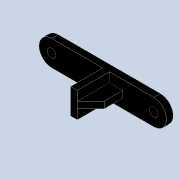
# Autodesk Inventor part: Y Axis Limit Switch Trigger
Saved by Autodesk Inventor 2022 (Build 260153000, 153)
## iProperties
Created: 2021-10-29
Part Number: Y Axis Limit Switch Trigger
Material: Generic
Document SubType Name: Modeling
Designer: Coy
Density: 1 g/cm^3
Appearance: Anodized - Black
Author: Coy
Autodesk Inventor part; units mm, degrees
ref_plane "YZ Plane" through (0, 0, 0) normal (1, 0, 0) x (0, 1, 0)
ref_plane "XZ Plane" through (0, 0, 0) normal (0, 1, 0) x (-1, 0, 0)
ref_plane "XY Plane" through (0, 0, 0) normal (0, 0, 1) x (1, 0, 0)
sketch "Sketch1" plane through (0, 0, 0) normal (0, 0, 1) x (1, 0, 0)
  circle A0 centre (0, 0) radius 3.175
  circle A1 centre (-76.2, 0) radius 3.175
  arc A2 (-76.2, 9.525) -> (-76.2, -9.525) centre (-76.2, 0) ccw
  arc A3 (0, -9.525) -> (0, 9.525) centre (0, 0) ccw
  line L0 (-76.2, 9.525) -> (0, 9.525)
  line L1 (-76.2, -9.525) -> (0, -9.525)
  dimension "d0" = 6.35
  dimension "d1" = 6.35
  dimension "d2" = 76.2
  dimension "d3" = 6.35
  dimension "d4" = 6.35
  constraints: 4 centre point, 4 end point, 4 point on circle, 2 tangent, 1 coincident
  measures "d0" diameter of A0
  measures "d1" diameter of A1
  measures "d2" distance of point (0, 0) A1.centre
  measures "d3" radial gap between concentric circles of A1 A2
  measures "d4" radial gap between concentric circles of A0 A3
extrude "Extrusion1" add sketch "Sketch1" along normal blind 5
sketch "Sketch2" plane through (0, 0, 5) normal (0, 0, 1) x (1, 0, 0)
  line L0 (0, 9.525) -> (-76.2, 9.525) projected
  line L1 (-76.2, -9.525) -> (0, -9.525) projected
  line L2 (-38.1, 9.525) -> (-33.1, 9.525)
  line L3 (-33.1, 9.525) -> (-33.1, -9.525)
  line L4 (-33.1, -9.525) -> (-38.1, -9.525)
  line L5 (-38.1, -9.525) -> (-38.1, 9.525)
  line L6 (-33.1, 2.5) -> (-23.1, 2.5)
  line L7 (-23.1, 2.5) -> (-23.1, -2.5)
  line L8 (-23.1, -2.5) -> (-33.1, -2.5)
  line L9 (-33.1, -2.5) -> (-33.1, 2.5)
  line L10 (-23.1, 0) -> (-38.1, 0) construction
  point P0 (0, 0)
  dimension "d7" = 5
  dimension "d8" = 10
  dimension "d9" = 5
  constraints: 18 end point, 4 parallel, 3 midpoint, 3 perpendicular, 2 horizontal, 2 point on line
  measures "d7" distance of L3.end L4.end
  measures "d8" distance of L7.end L8.end
  measures "d9" distance of L6.end L7.end
extrude "Extrusion2" add sketch "Sketch2" along normal blind 24
chamfer "Chamfer1" distance 10 angle 45 1 edges at (-23.1, 0, 29)
body "Solid1"
